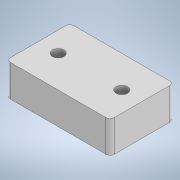
# Autodesk Inventor part: Teeth
Saved by Autodesk Inventor 2022 (Build 260153000, 153)
## iProperties
Created: 2021-11-02
Part Number: Teeth
Material: Genérico
Document SubType Name: Modeling
Designer: JK
Density: 1 g/cm^3
Appearance: Valor por defecto
Author: JK
Autodesk Inventor part; units mm, degrees
ref_plane "YZ Plane" through (0, 0, 0) normal (1, 0, 0) x (0, 1, 0)
ref_plane "XZ Plane" through (0, 0, 0) normal (0, 1, 0) x (-1, 0, 0)
ref_plane "XY Plane" through (0, 0, 0) normal (0, 0, 1) x (1, 0, 0)
sketch "Boceto1" plane through (0, 0, 0) normal (0, 1, 0) x (-1, 0, 0)
  line L0 (-24.5, 15) -> (24.5, 15)
  line L1 (24.5, 15) -> (24.5, -15)
  line L2 (24.5, -15) -> (-24.5, -15)
  line L3 (-24.5, -15) -> (-24.5, 15)
  line L4 (-24.5, 15) -> (24.5, -15) construction
  line L5 (24.5, 15) -> (-24.5, -15) construction
  point P0 (0, 0)
  dimension "d0" = 49
  dimension "d1" = 30
  constraints: 12 end point, 2 midpoint, 2 parallel, 1 horizontal, 1 perpendicular
  measures "d0" distance between parallel lines of L1 L3
  measures "d1" distance between parallel lines of L2 L0
extrude "Extrusión1" add sketch "Boceto1" along normal blind 15
sketch "Boceto2" plane through (0, 15, 0) normal (0, 1, 0) x (1, 0, 0)
  circle A0 centre (-15, 0) radius 2.7
  circle A1 centre (15, 0) radius 2.7
  line L0 (-24.5, 15) -> (-24.5, -15) projected
  line L1 (24.5, -15) -> (24.5, 15) projected
  point P0 (0, 0)
  dimension "d4" = 5.4
  dimension "d5" = 5.4
  dimension "d10" = 15
  dimension "d11" = 15
  constraints: 2 centre point, 2 horizontal alignment
  measures "d4" diameter of A0
  measures "d5" diameter of A1
  measures "d10" distance of A0.centre point (0, 0)
  measures "d11" distance of point (0, 0) A1.centre
extrude "Extrusión2" cut sketch "Boceto2" against normal blind 7.5
fillet "Empalme1" radius 2 4 edges at (-24.5, 7.5, 15) (24.5, 7.5, 15) (24.5, 7.5, -15) (-24.5, 7.5, -15)
